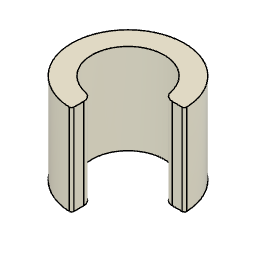
sample shifter spacer v1 (Autodesk Fusion 360 design; units mm, degrees)
Autodesk Fusion 360 part; units mm, degrees
sketch "Sketch1" plane through (0, 0, 0) normal (0, 1, 0) x (1, 0, 0)
  circle A0 centre (0, 0) radius 8
  circle A1 centre (0, 0) radius 12.5
  line L0 (0, 0) -> (12.5, 0)
  line L1 (0, 0) -> (0, -12.5)
  dimension "d1" = 16
  dimension "d2" = 25
  constraint coincident A0.centre A1.centre
  constraint concentric A0 A1
  constraint coincident A1 L0.end
  constraint horizontal L0
  constraint coincident A1 L1.end
  constraint perpendicular L0 L1
  measures "d1" diameter of A0
  measures "d2" diameter of A1
extrude "Extrude1" add sketch "Sketch1" along normal blind 20 contours A0 A1 L0 L1 picked at (-5.2365, -9.6417)
fillet "Fillet1" radius 2 2 edges at (8, 10, 0) (0, 10, 8)
fillet "Fillet2" radius 0.5 2 edges at (0, 10, 12.5) (12.5, 10, 0)
